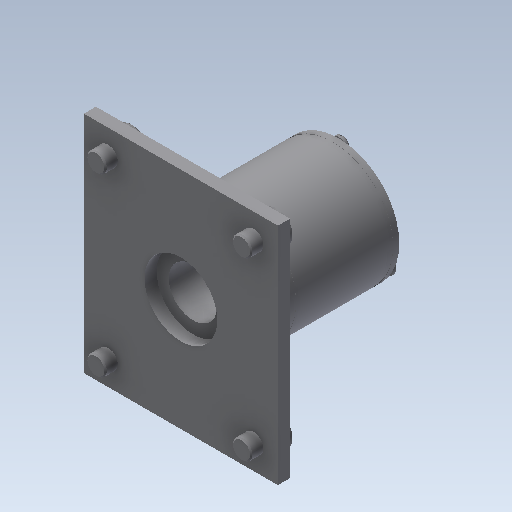
# Autodesk Inventor part: HTR3.7-7.5_J+H.9E4C23B774108A62587442637768E7FC
Saved by Autodesk Inventor 2021 (Build 250183000, 183)
## iProperties
Created: 2012-08-31
Material: Generic
Document SubType Name: Modeling
Designer: Parker Hannifin
Density: 1 g/cm^3
Part Number: HTR3.7-7.5_J+H.9E4C23B774108A62587442637768E7FC
Appearance: Default
Author: Parker Hannifin
Autodesk Inventor part; units mm, degrees
sketch "Sketch1" plane through (0, 0, 0) normal (1, 0, 0) x (0, 1, 0)
  line L0 (0, 16.51) -> (0, -99.06) construction
  line L1 (-6.35, 0) -> (38.1, 0) construction
  line L2 (19.05, 0) -> (19.05, -6.35)
  line L3 (19.05, -6.35) -> (12.7, -6.35)
  line L4 (12.7, -6.35) -> (12.7, -22.225)
  line L5 (12.7, -22.225) -> (1.6256, -22.225)
  line L6 (1.6256, -22.225) -> (1.6256, -24.384)
  line L7 (1.6256, -24.384) -> (3.0988, -24.384)
  line L8 (3.0988, -24.384) -> (3.0988, -26.67)
  line L9 (3.0988, -26.67) -> (9.5758, -26.67)
  line L10 (9.5758, -26.67) -> (9.5758, -28.575)
  line L11 (19.05, 0) -> (31.75, 0)
  line L12 (31.75, 0) -> (31.75, -28.5302)
  line L13 (31.75, -28.5302) -> (31.496, -28.575)
  line L14 (31.496, -28.575) -> (31.75, -28.6198)
  line L15 (31.75, -28.6198) -> (31.75, -79.3302)
  line L16 (31.75, -79.3302) -> (31.496, -79.375)
  line L17 (31.496, -79.375) -> (31.75, -79.4198)
  line L18 (31.75, -82.55) -> (0, -82.55)
  line L19 (9.5758, -28.575) -> (25.4, -28.575)
  line L20 (25.4, -28.575) -> (25.4, -79.375)
  line L21 (25.4, -79.375) -> (0, -79.375)
  line L22 (0, -82.55) -> (0, -79.375)
  line L23 (31.75, -79.4198) -> (31.75, -82.55)
  dimension "d1" = 19.05
  dimension "d3" = 12.7
  dimension "d4" = 1.6256
  dimension "d5" = 3.0988
  dimension "d6" = 9.5758
  dimension "d7" = 25.4
  dimension "d8" = 3.175
  dimension "d9" = 82.55
  dimension "d10" = 6.35
  dimension "d12" = 15.875
  dimension "d13" = 2.159
  dimension "d14" = 2.286
  dimension "d15" = 1.905
  dimension "d17" = 31.75
  dimension "d20" = 0.254
  dimension "d25" = 100
  dimension "d27" = 50.8
  dimension "d28" = 100
  constraints: 44 end point, 9 perpendicular, 6 parallel, 4 collinear, 3 point on line, 2 equal length
  measures "d1" distance between parallel lines of L2 L0
  measures "d3" distance between parallel lines of L0 L4
  measures "d4" distance between parallel lines of L0 L6
  measures "d5" distance between parallel lines of L0 L8
  measures "d6" distance between parallel lines of L0 L10
  measures "d7" distance between parallel lines of L0 L20
  measures "d8" distance between parallel lines of L18 L21
  measures "d9" distance between parallel lines of L18 L11
  measures "d10" distance between parallel lines of L3 L11
  measures "d12" distance between parallel lines of L5 L3
  measures "d13" distance between parallel lines of L7 L5
  measures "d14" distance between parallel lines of L9 L7
  measures "d15" distance between parallel lines of L9 L19
  measures "d17" distance between parallel lines of L0 L23
  measures "d20" distance from line of L13.end L12
  measures "d25" angle of L12 L13
  measures "d27" distance of L13.end L16.end
  measures "d28" angle of L15 L16
revolve "Revolution1" add sketch "Sketch1" angle 360 about axis through (0, 0, 0) along (0, 0, -1)
sketch "Sketch8" plane through (0, 0, 0) normal (0, 0, 1) x (1, 0, 0)
  line L0 (0, 44.45) -> (0, -44.45) construction
  line L1 (-44.45, 0) -> (44.45, 0) construction
  line L2 (-50.8, 58.801) -> (50.8, 58.801)
  line L3 (50.8, 58.801) -> (50.8, -58.801)
  line L4 (50.8, -58.801) -> (-50.8, -58.801)
  line L5 (-50.8, -58.801) -> (-50.8, 58.801)
  circle A0 centre (-38.1, 46.0375) radius 4.3688
  circle A1 centre (38.1, 46.0375) radius 4.3688
  circle A2 centre (38.1, -46.0375) radius 4.3688
  circle A3 centre (-38.1, -46.0375) radius 4.3688
  circle A4 centre (0, 0) radius 19.05 projected
  dimension "d77" = 117.602
  dimension "d78" = 101.6
  dimension "d79" = 76.2
  dimension "d80" = 92.075
  dimension "d81" = 8.7376
  constraints: 8 end point, 4 centre point, 3 equal radius, 2 horizontal alignment, 2 parallel, 2 symmetric about line, 2 vertical alignment, 1 horizontal, 1 perpendicular, 2 other
  measures "d77" distance of L2.end L3.end
  measures "d78" distance of L3.end L4.end
  measures "d79" distance of A1.centre A0.centre
  measures "d80" distance of A3.centre A0.centre
  measures "d81" diameter of A0
extrude "Extrusion7" add sketch "Sketch8" against normal blind 6.35
ref_plane "Work Plane3" through (0, -31.75, -53.975) normal (0, -1, 0) x (1, 0, 0)
sketch "Sketch7" plane through (0, -31.75, -53.975) normal (0, -1, 0) x (1, 0, 0)
  line L0 (0, -46.355) -> (0, 78.105) construction
  circle A0 centre (0, 0) radius 8.7376
  circle A1 centre (5.5372, 36.4998) radius 2.9718
  line L1 (-50.8, 53.975) -> (50.8, 53.975) construction
  dimension "d69" = 5.9436
  dimension "d70" = 17.4752
  dimension "d72" = 5.5372
  dimension "d84" = 17.4752
  dimension "d85" = 53.975
  constraints: 2 centre point, 1 point on line
  measures "d69" diameter of A1
  measures "d70" diameter of A0
  measures "d72" distance from line of A1.centre L0
  measures "d84" distance from line of A1.centre L1
  measures "d85" distance from line of A0.centre L1
extrude "Extrusion6" cut sketch "Sketch7" against normal blind 12.7
sketch "Sketch2" plane through (0, 0, -82.55) normal (0, 0, -1) x (-1, 0, 0)
  line L0 (0, -44.5821) -> (0, 45.2425) construction
  line L1 (-44.45, 0) -> (44.45, 0) construction
  circle A0 centre (0, 28.321) radius 4.0894
  circle A1 centre (24.5267, -14.1605) radius 4.0894
  circle A2 centre (-24.5267, -14.1605) radius 4.0894
  line L2 (24.5267, -14.1605) -> (0, 0) construction
  line L3 (0, 0) -> (-24.5267, -14.1605) construction
  dimension "d29" = 8.1788
  dimension "d30" = 28.321
  dimension "d31" = 28.321
  dimension "d32" = 120
  dimension "d33" = 120
  constraints: 4 end point, 3 centre point, 2 equal radius, 2 point on line, 1 equal length, 1 midpoint
  measures "d29" diameter of A0
  measures "d30" distance from line of L1 A0.centre
  measures "d31" distance of L2.start L2.end
  measures "d32" angle of L0 L2
  measures "d33" angle of L0 L3
extrude "Extrusion1" add sketch "Sketch2" along normal blind 2.4384
sketch "Sketch3" plane through (0, 28.321, -84.9884) normal (0, 0, -1) x (-1, 0, 0)
  circle A0 centre (0, 0) radius 4.0894 construction
  circle A1 centre (-24.5267, -42.4815) radius 4.0894 construction
  line L0 (0, -110.6424) -> (0, 54.0004) construction
  line L1 (-71.12, -28.321) -> (71.12, -28.321) construction
  line L2 (-0.6858, 6.35) -> (-0.6858, -6.35)
  line L3 (0.6858, 6.35) -> (0.6858, -6.35)
  line L4 (0.6858, -6.35) -> (-0.6858, -6.35)
  line L5 (0.6858, 6.35) -> (-0.6858, 6.35)
  line L6 (0, -28.321) -> (24.5267, -42.4815) construction
  line L7 (0, -28.321) -> (-24.5267, -42.4815) construction
  line L8 (23.8409, -36.1315) -> (23.8409, -48.8315)
  line L9 (25.2125, -36.1315) -> (25.2125, -48.8315)
  line L10 (25.2125, -36.1315) -> (23.8409, -36.1315)
  line L11 (23.8409, -48.8315) -> (25.2125, -48.8315)
  line L12 (-25.2125, -48.8315) -> (-25.2125, -36.1315)
  line L13 (-25.2125, -36.1315) -> (-23.8409, -36.1315)
  line L14 (-23.8409, -36.1315) -> (-23.8409, -48.8315)
  line L15 (-25.2125, -48.8315) -> (-23.8409, -48.8315)
  circle A2 centre (24.5267, -42.4815) radius 4.0894 construction
  line L16 (24.5267, -32.1725) -> (24.5267, -52.7905) construction
  line L17 (-24.5267, -32.1725) -> (-24.5267, -52.7905) construction
  dimension "d36" = 1.3716
  dimension "d37" = 12.7
  dimension "d38" = 6.35
  dimension "d39" = 1.3716
  dimension "d40" = 12.7
  dimension "d42" = 1.3716
  dimension "d43" = 12.7
  dimension "d48" = 6.35
  dimension "d49" = 6.35
  constraints: 32 end point, 7 perpendicular, 5 parallel, 4 midpoint, 1 coincident, 4 other
  measures "d36" distance between parallel lines of L3 L2
  measures "d37" distance of L3.start L3.end
  measures "d38" distance from line of L5 A0.centre
  measures "d39" distance between parallel lines of L8 L9
  measures "d40" distance of L9.start L9.end
  measures "d42" distance between parallel lines of L14 L12
  measures "d43" distance of L13.end L14.end
  measures "d48" distance from line of L10 A2.centre
  measures "d49" distance from line of L7.end L13
extrude "Extrusion2" cut sketch "Sketch3" against normal blind 1.4732
fillet "Fillet1" radius 1.3208 9 edges at (28.6161, -14.1605, -84.9884) (21.402, -16.7986, -84.9884) (21.402, -11.5224, -84.9884) (-3.1247, 25.6829, -84.9884) (-3.1247, 30.9591, -84.9884) (4.0894, 28.321, -84.9884) (-20.4373, -14.1605, -84.9884) (-27.6514, -16.7986, -84.9884) (-27.6514, -11.5224, -84.9884)
sketch "Sketch4" plane through (0, 0, -6.35) normal (0, 0, -1) x (-1, 0, 0)
  line L0 (-97.79, 0) -> (97.79, 0) construction
  circle A0 centre (0, 0) radius 19.05 construction
  circle A1 centre (-38.1, 46.0375) radius 8.255
  circle A2 centre (38.1, -46.0375) radius 8.255
  circle A3 centre (-38.1, -46.0375) radius 8.255
  circle A4 centre (38.1, 46.0375) radius 4.3688 construction
  circle A5 centre (-38.1, 46.0375) radius 4.3688 construction
  circle A6 centre (-38.1, -46.0375) radius 4.3688 construction
  circle A7 centre (38.1, -46.0375) radius 4.3688 construction
  circle A8 centre (38.1, 46.0375) radius 8.255
  dimension "d51" = 16.51
  constraints: 5 centre point, 4 coincident, 3 equal radius, 2 end point
  measures "d51" diameter of A1
extrude "Extrusion3" add sketch "Sketch4" along normal blind 6.35
sketch "Sketch5" plane through (38.1, 46.0375, -12.7) normal (0, 0, -1) x (-1, 0, 0)
  line L0 (0, -4.3994) -> (-3.81, -2.1997)
  line L1 (-3.81, -2.1997) -> (-3.81, 2.1997)
  line L2 (-3.81, 2.1997) -> (0, 4.3994)
  line L3 (0, 4.3994) -> (3.81, 2.1997)
  line L4 (3.81, 2.1997) -> (3.81, -2.1997)
  line L5 (3.81, -2.1997) -> (0, -4.3994)
  line L6 (76.2, -96.4744) -> (72.39, -94.2747)
  line L7 (72.39, -94.2747) -> (72.39, -89.8753)
  line L8 (72.39, -89.8753) -> (76.2, -87.6756)
  line L9 (76.2, -87.6756) -> (80.01, -89.8753)
  line L10 (80.01, -89.8753) -> (80.01, -94.2747)
  line L11 (80.01, -94.2747) -> (76.2, -96.4744)
  line L12 (0, -96.4744) -> (-3.81, -94.2747)
  line L13 (-3.81, -94.2747) -> (-3.81, -89.8753)
  line L14 (-3.81, -89.8753) -> (0, -87.6756)
  line L15 (0, -87.6756) -> (3.81, -89.8753)
  line L16 (3.81, -89.8753) -> (3.81, -94.2747)
  line L17 (3.81, -94.2747) -> (0, -96.4744)
  circle A0 centre (76.2, 0) radius 8.255 construction
  circle A1 centre (0, 0) radius 8.255 construction
  circle A2 centre (0, -92.075) radius 8.255 construction
  circle A3 centre (76.2, -92.075) radius 8.255 construction
  line L18 (76.2, -4.3994) -> (72.39, -2.1997)
  line L19 (72.39, -2.1997) -> (72.39, 2.1997)
  line L20 (72.39, 2.1997) -> (76.2, 4.3994)
  line L21 (76.2, 4.3994) -> (80.01, 2.1997)
  line L22 (80.01, 2.1997) -> (80.01, -2.1997)
  line L23 (80.01, -2.1997) -> (76.2, -4.3994)
  line L24 (38.1, -128.3589) -> (38.1, 36.2839) construction
  line L25 (-33.02, -46.0375) -> (109.22, -46.0375) construction
  dimension "d56" = 7.62
  dimension "d57" = 7.62
  dimension "d58" = 7.62
  dimension "d86" = 7.62
  constraints: 48 end point, 4 coincident, 4 parallel, 52 other
  measures "d56" distance between parallel lines of L1 L4
  measures "d57" distance between parallel lines of L16 L13
  measures "d58" distance between parallel lines of L10 L7
  measures "d86" distance from line of L22.end L19
extrude "Extrusion4" cut sketch "Sketch5" against normal blind 4.064
sketch "Sketch6" plane through (-50.8, 58.801, 0) normal (0, 0, 1) x (1, 0, 0)
  circle A0 centre (88.9, -12.7635) radius 5.08
  circle A1 centre (12.7, -104.8385) radius 5.08
  circle A2 centre (88.9, -104.8385) radius 5.08
  circle A3 centre (12.7, -12.7635) radius 5.08
  circle A4 centre (88.9, -12.7635) radius 4.3688 construction
  circle A5 centre (88.9, -104.8385) radius 4.3688 construction
  circle A6 centre (12.7, -104.8385) radius 4.3688 construction
  circle A7 centre (12.7, -12.7635) radius 4.3688 construction
  dimension "d61" = 10.16
  constraints: 4 centre point, 4 coincident, 3 equal radius
  measures "d61" diameter of A0
extrude "Extrusion5" add sketch "Sketch6" along normal blind 6.35
chamfer "Chamfer1" distance 0.635 angle 45 8 edges at (33.02, 46.0375, 6.35) (-43.18, -46.0375, 6.35) (33.02, -46.0375, 6.35) (46.355, -46.0375, -12.7) (46.355, 46.0375, -12.7) (-29.845, -46.0375, -12.7) (-43.18, 46.0375, 6.35) (-29.845, 46.0375, -12.7)
ref_plane "WP_Housing-REAR" through (-50.8, 58.801, 0) normal (0, 0, 1) x (1, 0, 0)
ref_plane "WP_H" through (0, 0, 0) normal (0, -1, 0) x (1, 0, 0)
body "Solid1"
